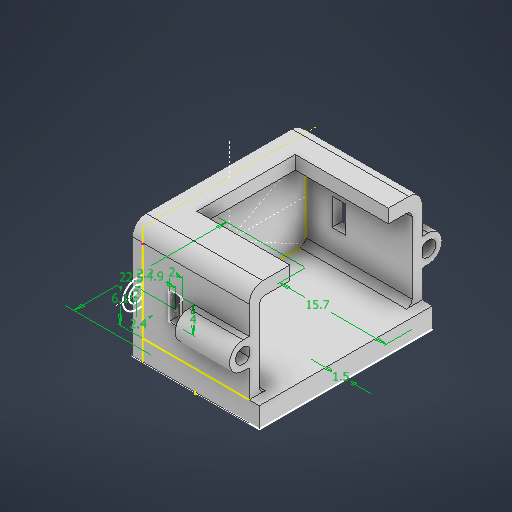
# Autodesk Inventor part: Horizontal_Servo_Adapter
Saved by Autodesk Inventor 2026.1 (Build 301233000, 233)
## iProperties
Created: 2026-03-10
Part Number: Horizontal_Servo_Adapter
Material: Generic
Document SubType Name: Modeling
Designer: WinFlame
Density: 1 g/cm^3
Appearance: Default
Project: Myoelectric_Arm
Author: WinFlame
Autodesk Inventor part; units mm, degrees
ref_plane "YZ Plane" through (0, 0, 0) normal (1, 0, 0) x (0, 1, 0)
ref_plane "XZ Plane" through (0, 0, 0) normal (0, 1, 0) x (-1, 0, 0)
ref_plane "XY Plane" through (0, 0, 0) normal (0, 0, 1) x (1, 0, 0)
sketch "Master Sketch" plane through (0, 0, -46.0496) normal (0, 1, 0) x (-1, 0, 0)
  line L0 (7.85, 57.2996) -> (-7.85, 57.2996)
  line L1 (-7.85, 57.2996) -> (-7.85, 34.7996)
  line L2 (-7.85, 34.7996) -> (7.85, 34.7996)
  line L3 (7.85, 34.7996) -> (7.85, 57.2996)
  line L4 (7.85, 57.2996) -> (-7.85, 34.7996) construction
  line L5 (-7.85, 57.2996) -> (7.85, 34.7996) construction
  line L6 (-9.35, 33.2996) -> (-9.35, 58.7996)
  line L7 (-9.35, 58.7996) -> (9.35, 58.7996)
  line L8 (9.35, 58.7996) -> (9.35, 33.2996)
  line L9 (9.35, 33.2996) -> (-9.35, 33.2996)
  line L10 (-7.85, 57.2996) -> (-9.35, 57.2996) construction
  line L11 (-7.85, 34.7996) -> (-9.35, 34.7996) construction
  line L12 (-7.85, 34.7996) -> (-7.85, 33.2996)
  line L13 (-7.85, 57.2996) -> (-7.85, 58.7996)
  point P0 (0, 46.0496)
  point P1 (0, 46.0496)
  dimension "d3" = 22.5
  dimension "d0" = 1.5
  dimension "d30" = 15.7
  constraints: 28 end point, 5 perpendicular, 5 point on line, 4 parallel, 2 coincident, 2 horizontal, 2 midpoint, 3 other
  measures "d3" distance of L2.end L0.start
  measures "d0" distance between parallel lines of L1 L6
  measures "d30" distance of L1.end L2.end
extrude "BasePlate Extrude" add sketch "Master Sketch" along normal blind 3
extrude "Walls Extrude" add sketch "Master Sketch" along normal blind 12.2 from surface at 3 contours L0 L13 L7 L8 L9 L12 L2 L3
extrude "Roof Extrude" add sketch "Master Sketch" along normal blind 2 from surface at 15.2 contours L3 L2 L1 L0 | L0 L13 L7 L8 L9 L12 L2 L3
sketch "Reference Sketch" plane through (-7.85, 3, 11.25) normal (1, 0, 0) x (0, 0, -1)
  line L0 (22.5, 0) -> (0, 0)
  line L1 (0, 0) -> (0, 12.2)
  line L2 (0, 12.2) -> (22.5, 12.2)
  line L3 (22.5, 12.2) -> (22.5, 0)
  line L4 (22.5, 0) -> (0, 12.2) construction
  line L5 (0, 0) -> (22.5, 12.2) construction
  line L6 (0, 0) -> (0, 12.2) projected
  line L7 (24, 12.2) -> (-1.5, 12.2) projected
  line L8 (-1.5, 0) -> (24, 0) projected
  line L9 (22.5, 12.2) -> (22.5, 0) projected
  line L10 (-5.714, 6.1) -> (28.214, 6.1) construction
  line L11 (-1.5, 5.1) -> (-1.5, 7.1)
  line L12 (-1.5, -3) -> (-1.5, 14.2) projected
  circle A0 centre (-2.4, 6.1) radius 1.1
  arc A1 (-2.4, 8.1) -> (-2.4, 4.1) centre (-2.4, 6.1) ccw
  line L13 (-2.4, 8.1) -> (-1.5, 8.1)
  line L14 (-2.4, 4.1) -> (-1.5, 4.1)
  line L15 (-1.5, 8.1) -> (-1.5, 4.1)
  line L16 (11.25, -6.8706) -> (11.25, 19.0706) construction
  line L17 (-1.5, 14.2) -> (24, 14.2) construction
  line L18 (24, 5.1) -> (24, 7.1)
  circle A2 centre (24.9, 6.1) radius 1.1
  arc A3 (24.9, 4.1) -> (24.9, 8.1) centre (24.9, 6.1) ccw
  line L19 (24.9, 8.1) -> (24, 8.1)
  line L20 (24.9, 4.1) -> (24, 4.1)
  line L21 (24, 8.1) -> (24, 4.1)
  point P0 (11.25, -3)
  point P1 (11.25, 6.1)
  point P2 (-1.5, 6.1)
  point P3 (24, 6.1)
  point P4 (24, 7.1)
  dimension "d38" = 2.2
  dimension "d55" = 2
  dimension "d56" = 180
  dimension "d57" = 2.4
  constraints: 32 end point, 9 symmetric about line, 6 point on line, 5 midpoint, 4 centre point, 4 perpendicular, 4 point on circle, 3 horizontal, 2 coincident, 2 parallel, 1 vertical, 1 vertical alignment, 6 other
  measures "d38" diameter of A0
  measures "d55" radius of A1
  measures "d57" distance from line of A0.centre L1
fillet "Fillet1" radius 0.85 4 edges at (0, 3, 11.25) (0, 15.2, 11.25) (0, 3, -11.25) (0, 15.2, -11.25)
fillet "Fillet1" radius 2 2 edges at (-0.75, 17.2, 12.75) (-0.75, 17.2, -12.75)
extrude "Screw Holes" add sketch "Reference Sketch" against normal blind 6 from surface at 15.7 contours L14 A1 L13 L12 L11 A0 | L18 A2 L21 L19 A3 L20
sketch "Sketch7" plane through (-9.35, 0, 12.75) normal (0, 0, 1) x (1, 0, 0)
  line L0 (5.4, 7.1) -> (7.4, 7.1)
  line L1 (7.4, 7.1) -> (7.4, 11.1)
  line L2 (7.4, 11.1) -> (5.4, 11.1)
  line L3 (5.4, 11.1) -> (5.4, 7.1)
  line L4 (5.4, 7.1) -> (7.4, 11.1) construction
  line L5 (7.4, 7.1) -> (5.4, 11.1) construction
  line L6 (17.2, 3) -> (1.5, 3) projected
  line L7 (1.5, 3.85) -> (1.5, 14.35) projected
  point P0 (9.35, 0)
  point P1 (6.4, 9.1)
  dimension "d48" = 2
  dimension "d49" = 4
  dimension "d50" = 6.1
  dimension "d51" = 4.9
  constraints: 12 end point, 2 midpoint, 2 parallel, 1 horizontal, 1 perpendicular
  measures "d48" distance of L2.end L1.end
  measures "d49" distance of L1.end L0.end
  measures "d50" distance from line of L6 point (6.4, 9.1)
  measures "d51" distance from line of L7 point (6.4, 9.1)
extrude "Holes for Wire" cut sketch "Sketch7" against normal up to surface (25.5 mm away)
sketch "Sketch9" plane through (-9.35, 17.2, -10.75) normal (0, 1, 0) x (1, 0, 0)
  line L0 (18.7, -23.5) -> (18.7, 2) projected
  line L1 (3.5, -17.5) -> (18.7, -17.5)
  line L2 (18.7, -17.5) -> (18.7, -3)
  line L3 (18.7, -3) -> (3.5, -3)
  line L4 (3.5, -3) -> (3.5, -17.5)
  line L5 (17.2, -21.5) -> (0, -21.5) projected
  line L6 (1.5, -0.35) -> (1.5, -21.15) projected
  line L7 (0, 0) -> (17.2, 0) projected
  point P0 (9.35, -10.75)
  point P1 (18.7, -21.5)
  point P2 (18.7, 0)
  dimension "d58" = 4
  dimension "d59" = 2
  dimension "d60" = 3
  constraints: 8 end point, 2 parallel, 1 horizontal, 1 perpendicular, 1 point on line
  measures "d58" distance between parallel lines of L5 L1
  measures "d59" distance between parallel lines of L6 L4
  measures "d60" distance between parallel lines of L7 L3
extrude "Extrusion10" cut sketch "Sketch9" against normal up to surface (2 mm away)
extrude "Extrusion11" add sketch "Reference Sketch" against normal blind 2 from surface at 9.7 contours L14 A1 L13 L12 L11 A0 | A0 L11 | L18 A2 L21 L19 A3 L20 | L18 A2 picked at (-2.0439, 5.8262) picked at (24.6286, 6.2627)
body "Solid1"
